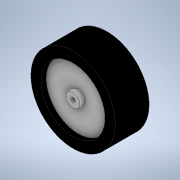
# Autodesk Inventor part: roda
Saved by Autodesk Inventor 2020 (Build 240168000, 168)
## iProperties
Created: 2020-04-18
Part Number: roda
Material: Genérico
Document SubType Name: Modeling
Designer: eduardoADM
Density: 1 g/cm^3
Appearance: Padrão
Author: eduardoADM
Autodesk Inventor part; units mm, degrees
ref_plane "YZ Plane" through (0, 0, 0) normal (1, 0, 0) x (0, 1, 0)
ref_plane "XZ Plane" through (0, 0, 0) normal (0, 1, 0) x (-1, 0, 0)
ref_plane "XY Plane" through (0, 0, 0) normal (0, 0, 1) x (1, 0, 0)
sketch "Esboço2" plane through (0, 0, 0) normal (0, 0, 1) x (1, 0, 0)
  circle A0 centre (0, 0) radius 33
  dimension "d5" = 66
  constraints: 1 centre point, 1 coincident
  measures "d5" diameter of A0
extrude "Extrusão2" add sketch "Esboço2" along normal blind 26.6
sketch "Esboço9" plane through (0, 0, 26.6) normal (0, 0, 1) x (1, 0, 0)
  circle A0 centre (0, 0) radius 25
  dimension "d18" = 50
  constraints: 1 centre point, 1 coincident
  measures "d18" diameter of A0
extrude "Extrusão5" cut sketch "Esboço9" against normal blind 4
sketch "Esboço12" plane through (0, 0, 22.6) normal (0, 0, 1) x (1, 0, 0)
  circle A0 centre (0, 0) radius 5.4
  dimension "d24" = 10.8
  constraints: 1 centre point, 1 coincident
  measures "d24" diameter of A0
extrude "Extrusão7" add sketch "Esboço12" along normal blind 4
sketch "Esboço13" plane through (0, 0, 26.6) normal (0, 0, 1) x (1, 0, 0)
  circle A0 centre (0, 0) radius 1.8
  dimension "d27" = 3.6
  constraints: 1 centre point, 1 coincident
  measures "d27" diameter of A0
extrude "Extrusão8" cut sketch "Esboço13" against normal through all
ref_plane "Plano de trabalho1" through (0, 0, 13.3) normal (0, 0, 1) x (1, 0, 0)
mirror "Espelhamento2" about plane through (0, 0, 13.3) normal (0, 0, 1) of "Extrusão8", "Extrusão7", "Extrusão5"
